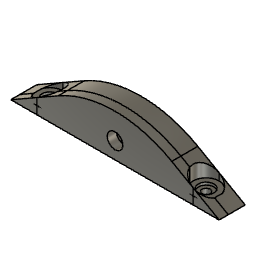
bearingholder (Autodesk Fusion 360 design; units mm, degrees)
Autodesk Fusion 360 part; units mm, degrees
form "フォーム1" [no effect]
sketch "スケッチ1" plane through (0, 0, 0) normal (0, 0, 1) x (1, 0, 0)
  line L0 (0, 0) -> (80, 0)
  line L1 (80, 0) -> (80, 5)
  line L2 (80, 5) -> (0, 5)
  line L3 (0, 5) -> (0, 0)
  circle A0 centre (10, 2.5) radius 1.5
  circle A1 centre (10, 2.5) radius 5
  circle A2 centre (10, 2.5) radius 3
  circle A3 centre (70, 2.5) radius 5
  circle A4 centre (70, 2.5) radius 3
  circle A5 centre (70, 2.5) radius 1.5
  constraint horizontal L0
  constraint vertical L1
  constraint horizontal L2
  constraint vertical L3
  constraint coincident L0.start L3.end
  constraint concentric A0 A1
  constraint concentric A1 A2
extrude "押し出し1" add sketch "スケッチ1" along normal blind 2 contours L0 L2 L3 A1 | L0 L2 A2 | L0 A2 | L0 L2 A1 A3 | L2 A2 | L0 L2 A4 | L0 A4 | L0 L1 L2 A3 | L2 A4 makes body 1 at (48.338, 2.3754, 0) makes body 2 at (78.3287, 2.6246, 2) makes body 3 at (12.9963, 2.3505, 0.6667) makes body 4 at (69.627, 5.4767, 0.6667) makes body 5 at (1.6713, 2.6246, 0)
extrude "押し出し2" add sketch "スケッチ1" along normal blind 20 contours L0 L2 A1 A2 | L0 A1 A2 | L2 A1 A2 | L0 L2 A1 A2 | L0 L2 A3 A4 | L0 A3 A4 | L2 A3 A4 | L0 L2 A3 A4 bodies 1 2 3 4 5
extrude "押し出し3" add 3 faces at (48.3427, 2.5, 2) (78.3333, 2.5, 2) (1.6713, 2.6246, 2) along direction (0, 0, 1) blind 30 on bodies 1 bodies 1
sketch "スケッチ2" plane through (0, 0, 0) normal (0, -1, 0) x (1, 0, 0)
  line L0 (14.3301, 0) -> (65.6699, 0)
  line L1 (65.6699, 0) -> (65.6699, 20)
  line L2 (65.6699, 20) -> (65.6699, 32)
  line L3 (65.6699, 32) -> (14.3301, 32)
  line L4 (14.3301, 32) -> (14.3301, 20)
  line L5 (14.3301, 20) -> (14.3301, 0)
  line L6 (0, 0) -> (35.0031, 20)
  line L7 (45, 20) -> (80, 0)
  arc A0 (45, 20) -> (35.0031, 20) centre (40.0016, 11.252) ccw
  line L8 (0, 0) -> (80.0579, 0)
  line L9 (80.0579, 0) -> (80.0579, 32)
  line L10 (80.0579, 32) -> (0, 32)
  line L11 (0, 32) -> (0, 0)
  constraint coincident L6.start L8.start
  constraint tangent L6 A0
  constraint horizontal L8
  constraint vertical L9
  constraint horizontal L10
  constraint vertical L11
extrude "押し出し4" cut sketch "スケッチ2" along normal mid plane 20 contours L4 L5 L6 L10 L11 | L1 L2 L3 L4 L5 L6 L7 A0 L10 | L1 L2 L7 L8 L9 L10 bodies 1
sketch "スケッチ3" plane through (0, 0, 0) normal (0, -1, 0) x (1, 0, 0)
  line L0 (35.0031, 20) -> (14.3301, 8.1879)
  line L1 (14.3301, 8.1879) -> (14.3301, 0)
  line L2 (14.3301, 0) -> (65.6699, 0)
  line L3 (65.6699, 0) -> (65.6699, 8.1886)
  line L4 (65.6699, 8.1886) -> (45, 20)
  arc A0 (45, 20) -> (35.0031, 20) centre (40.0016, 11.252) ccw
  line L5 (40.0016, 21.3273) -> (40.0016, 0)
  line L6 (40.0016, 0) -> (40.0016, 6.35)
  circle A1 centre (40.0016, 6.35) radius 5
  dimension "d9" = 6.35
  dimension "d10" = 10
  constraint midpoint A0 L5.start
  constraint vertical L5
  constraint perpendicular L2 L6
  constraint coincident L6.end A1.centre
  measures "d9" distance of L5.end L6.end
  measures "d10" diameter of A1
extrude "押し出し5" cut sketch "スケッチ3" against normal blind 21 contours L5 L6 A1 | L5 L6 A1 bodies 1
extrude "押し出し6" cut 3 faces at (28.2767, 0, 12.2358) (76.2201, 0, 1.08) (3.7799, 0, 1.0799) along direction (0, 1, 0) blind 1 on bodies 1 bodies 1
extrude "押し出し7" cut 3 faces at (28.2767, 5, 12.2358) (76.2201, 5, 1.08) (3.7799, 5, 1.0799) along direction (0, -1, 0) blind 1 on bodies 1 bodies 1
extrude "押し出し8" add sketch "スケッチ1" along normal blind 16 contours L0 L2 A1 A2 | L0 A1 A2 | L2 A1 A2 | L0 L2 A1 A2 bodies 1
extrude "押し出し9" add sketch "スケッチ1" along normal blind 17 contours L0 L2 A3 A4 | L0 A3 A4 | L2 A3 A4 | L0 L2 A3 A4 bodies 1
extrude "押し出し10" cut sketch "スケッチ2" along normal mid plane 28 contours L4 L5 L6 L10 L11 | L1 L2 L3 L4 L5 L6 L7 A0 L10 | L1 L2 L7 L8 L9 L10 bodies 1
extrude "押し出し11" add sketch "スケッチ1" along normal blind 15 contours L0 L2 A3 A4 | L0 A3 A4 | L2 A3 A4 | L0 L2 A3 A4 bodies 1
extrude "押し出し12" cut 1 faces at (68.0578, -1.3609, 15) along direction (0, 0, -1) blind 12 on bodies 1 bodies 1
sketch "スケッチ4" plane through (0, 0, 3) normal (0, 0, 1) x (-1, 0, 0)
  circle A0 centre (-70, -2.5) radius 3
  arc A1 (-65.2303, -4) -> (-65.2303, -1) centre (-70, -2.5) ccw
  arc A2 (-65.2303, -1) -> (-65.2303, -4) centre (-70, -2.5) ccw
  line L0 (-65.2303, -4) -> (-67.4019, -4)
  line L1 (-65.2303, -1) -> (-67.4019, -1)
  constraint coincident A1.start A2.end
  constraint coincident A0 L0.end
  constraint horizontal L0
  constraint coincident A1.end A2.start
  constraint coincident A0 L1.end
  constraint parallel L0 L1
extrude "押し出し13" add sketch "スケッチ4" along normal blind 6 contours A0 A1 L0 L1 bodies 1
extrude "押し出し14" cut sketch "スケッチ2" against normal blind 30 contours L1 L2 L3 L4 L5 L6 L7 A0 L10 | L1 L2 L7 L8 L9 L10 bodies 1
extrude "押し出し15" add sketch "スケッチ1" along normal blind 13 contours L0 L2 A1 A2 | L0 A1 A2 | L2 A1 A2 | L0 L2 A1 A2 bodies 1
extrude "押し出し16" cut 1 faces at (14.3147, 2.7484, 13) along direction (0, 0, -1) blind 10 on bodies 1 bodies 1
sketch "スケッチ5" plane through (0, 0, 3) normal (0, 0, 1) x (-1, 0, 0)
  circle A0 centre (-10, -2.5) radius 3
  arc A1 (-14.7697, -4) -> (-14.7697, -1) centre (-10, -2.5) ccw
  arc A2 (-14.7697, -1) -> (-14.7697, -4) centre (-10, -2.5) ccw
  line L0 (-14.7697, -4) -> (-12.5981, -4)
  line L1 (-14.7697, -1) -> (-12.5981, -1)
  constraint coincident A1.start A2.end
  constraint coincident A0 L0.end
  constraint horizontal L0
  constraint coincident A1.end A2.start
  constraint coincident A0 L1.end
  constraint parallel L0 L1
extrude "押し出し17" add sketch "スケッチ5" along normal blind 8 contours A0 A2 L0 L1 bodies 1
extrude "押し出し18" cut sketch "スケッチ2" against normal blind 13 contours L4 L5 L6 L10 L11 | L1 L2 L3 L4 L5 L6 L7 A0 L10 bodies 1
copy_body "ボディ -> コンポーネント1" bodies 1 removing the originals makes body 6 in component "Component'"
sketch "スケッチ6" plane through (0, 1, 0) normal (0, -1, 0) x (1, 0, 0)
  line L0 (35.0031, 20) -> (12.5981, 7.1983)
  line L1 (12.5981, 7.1983) -> (12.5981, 3)
  line L2 (12.5981, 3) -> (14.7697, 3)
  line L3 (14.7697, 3) -> (14.7697, 0)
  line L4 (14.7697, 0) -> (65.2303, 0)
  line L5 (65.2303, 0) -> (65.2303, 3)
  line L6 (65.2303, 3) -> (67.4019, 3)
  line L7 (67.4019, 3) -> (67.4019, 7.1989)
  line L8 (67.4019, 7.1989) -> (45, 20)
  arc A0 (45, 20) -> (35.0031, 20) centre (40.0016, 11.252) ccw
  circle A1 centre (40.0016, 6.35) radius 5
  line L9 (12.5981, 7.1983) -> (23.8006, 13.5991)
  line L10 (18.1993, 10.3987) -> (12.5981, 7.1983)
  line L11 (67.4019, 7.1989) -> (56.201, 13.5995)
  line L12 (61.8014, 10.3992) -> (67.4019, 7.1989)
  arc A2 (61.8014, 10.3992) -> (18.1993, 10.3987) centre (40.0008, -27.7573) ccw
  constraint coincident L0.end L1.start
  constraint midpoint L0 L9.end
  constraint midpoint L9 L10.start
  constraint coincident L7.end L8.start
  constraint midpoint L8 L11.end
  constraint midpoint L11 L12.start
  constraint tangent L10 A2
extrude "押し出し1'" cut sketch "スケッチ6" against normal blind 30 contours L0 L8 A0 L9 L11 A2 bodies 6 in component "Component'"
sketch "スケッチ7" plane through (0, 0, 0) normal (0, 0, -1) x (1, 0, 0)
  circle A0 centre (70, -2.5) radius 1.5
  line L0 (14.7697, -4) -> (65.2303, -4)
  arc A1 (65.2303, -4) -> (74.7697, -4) centre (70, -2.5) ccw
  line L1 (74.7697, -4) -> (80, -4)
  line L2 (80, -4) -> (80, -1)
  line L3 (80, -1) -> (74.7697, -1)
  arc A2 (74.7697, -1) -> (65.2303, -1) centre (70, -2.5) ccw
  line L4 (65.2303, -1) -> (14.7697, -1)
  arc A3 (14.7697, -1) -> (5.2303, -1) centre (10, -2.5) ccw
  line L5 (5.2303, -1) -> (0, -1)
  line L6 (0, -1) -> (0, -4)
  line L7 (0, -4) -> (5.2303, -4)
  arc A4 (5.2303, -4) -> (14.7697, -4) centre (10, -2.5) ccw
  circle A5 centre (10, -2.5) radius 1.5
  line L8 (10, 2.5) -> (70, 2.5)
  line L9 (70, 2.5) -> (80, 2.5)
  line L10 (80, -1) -> (80, 2.5)
  line L11 (10, 2.5) -> (0, 2.5)
  line L12 (0, 2.5) -> (0, -1)
  constraint midpoint A3 L8.start
  constraint midpoint A2 L8.end
  constraint tangent A2 L9
  constraint parallel L8 L9
  constraint coincident L2.end L3.start
  constraint perpendicular L9 L10
  constraint tangent A3 L11
  constraint perpendicular L10 L11
  constraint coincident L5.end L6.start
  constraint perpendicular L5 L12
extrude "押し出し19" add sketch "スケッチ7" against normal blind 18 separate body contours A3 L5 L11 L12 | L3 A2 L9 L10 | A2 L4 A3 L8 makes body 7
sketch "スケッチ8" plane through (0, 4, 0) normal (0, 1, 0) x (-1, 0, 0)
  arc A0 (-18.1993, 10.3987) -> (-61.8014, 10.3992) centre (-40.0008, -27.7573) ccw
  line L0 (-61.8014, 10.3992) -> (-67.4019, 7.1989)
  line L1 (-67.4019, 7.1989) -> (-67.4019, 3)
  line L2 (-67.4019, 3) -> (-65.2303, 3)
  line L3 (-65.2303, 3) -> (-65.2303, 0)
  line L4 (-65.2303, 0) -> (-14.7697, 0)
  line L5 (-14.7697, 0) -> (-14.7697, 3)
  line L6 (-14.7697, 3) -> (-12.5981, 3)
  line L7 (-12.5981, 3) -> (-12.5981, 7.1983)
  line L8 (-12.5981, 7.1983) -> (-18.1993, 10.3987)
  circle A1 centre (-40.0016, 6.35) radius 5
  line L9 (0, 0) -> (0, 18)
  line L10 (0, 18) -> (-80, 18)
  line L11 (-80, 18) -> (-80, 0)
  line L12 (-80, 0) -> (0, 0)
  line L13 (-61.8014, 10.3992) -> (-80, 0)
  line L14 (0, 0) -> (-18.1993, 10.3987)
  arc A2 (-18.1993, 10.3987) -> (-61.8014, 10.3992) centre (-40.0008, -27.7573) ccw
  constraint coincident L9.start L12.end
  constraint perpendicular L6 L9
  constraint perpendicular L7 L10
  constraint perpendicular L10 L11
  constraint perpendicular L9 L12
  constraint coincident A0.end L0.start
  constraint coincident A0.start L8.end
  constraint tangent L14 A2
extrude "押し出し20" cut sketch "スケッチ8" against normal blind 11 contours A0 L0 L8 L9 L10 L11 L13 L14 A2 bodies 7
extrude "押し出し2'" add 1 faces at (74.1667, 2.5, 3) along direction (0, 0, 1) blind 6 on bodies 6 bodies 6 in component "Component'"
sketch "スケッチ9" plane through (0, 0, 9) normal (0, 0, 1) x (-1, 0, 0)
  line L0 (-74.75, -0.9388) -> (-74.75, -4.0612)
  arc A0 (-74.75, -4.0612) -> (-65.2303, -4) centre (-70, -2.5) ccw
  line L1 (-65.2303, -4) -> (-67.4019, -4)
  arc A1 (-67.4019, -1) -> (-67.4019, -4) centre (-70, -2.5) ccw
  line L2 (-67.4019, -1) -> (-65.2303, -1)
  arc A2 (-65.2303, -1) -> (-74.75, -0.9388) centre (-70, -2.5) ccw
  circle A3 centre (-70, -2.5) radius 5
  circle A4 centre (-70, -2.5) radius 3
  dimension "d47" = 10
  dimension "d48" = 6
  constraint concentric A0 A3
  constraint concentric A0 A4
  measures "d47" diameter of A3
  measures "d48" diameter of A4
extrude "押し出し3'" cut sketch "スケッチ9" against normal blind 6 contours L0 A0 L1 A1 L2 A2 A3 A4 | L0 A3 | L1 L2 A3 A4 bodies 6 in component "Component'"
extrude "押し出し4'" add 1 faces at (5.8364, 2.4253, 3) along direction (0, 0, 1) blind 6 on bodies 6 bodies 6 in component "Component'"
sketch "スケッチ10" plane through (0, 0, 9) normal (0, 0, 1) x (-1, 0, 0)
  line L0 (-5.2505, -4.0627) -> (-5.2505, -0.9373)
  arc A0 (-5.2505, -0.9373) -> (-14.7697, -1) centre (-10, -2.5) ccw
  line L1 (-14.7697, -1) -> (-12.5981, -1)
  arc A1 (-12.5981, -4) -> (-12.5981, -1) centre (-10, -2.5) ccw
  line L2 (-12.5981, -4) -> (-14.7697, -4)
  arc A2 (-14.7697, -4) -> (-5.2505, -4.0627) centre (-10, -2.5) ccw
  circle A3 centre (-10, -2.5) radius 3
  circle A4 centre (-10, -2.5) radius 5
  dimension "d53" = 6
  dimension "d54" = 10
  constraint concentric A0 A3
  constraint concentric A3 A4
  measures "d53" diameter of A3
  measures "d54" diameter of A4
extrude "押し出し5'" cut sketch "スケッチ10" against normal blind 6 contours L0 A0 L1 A1 L2 A2 A3 A4 | L0 A4 | L1 L2 A3 A4 bodies 6 in component "Component'"
sketch "スケッチ11" plane through (0, 4, 0) normal (0, 1, 0) x (-1, 0, 0)
  line L0 (-14.7697, 0) -> (-14.7697, 3)
  line L1 (-14.7697, 3) -> (-14.7697, 8.4391)
  line L2 (-14.7697, 8.4391) -> (-18.1993, 10.3987)
  arc A0 (-18.1993, 10.3987) -> (-61.8014, 10.3992) centre (-40.0008, -27.7573) ccw
  line L3 (-61.8014, 10.3992) -> (-65.2303, 8.4398)
  line L4 (-65.2303, 8.4398) -> (-65.2303, 3)
  line L5 (-65.2303, 3) -> (-65.2303, 0)
  line L6 (-65.2303, 0) -> (-14.7697, 0)
  circle A1 centre (-40.0016, 6.35) radius 5
  circle A2 centre (-40.0016, 6.35) radius 5
  dimension "d57" = 10
  constraint concentric A1 A2
  measures "d57" diameter of A2
extrude "押し出し21" cut sketch "スケッチ11" against normal blind 10 contours A1 A2 bodies 7
sketch "スケッチ12" plane through (0, 4, 0) normal (0, 1, 0) x (-1, 0, 0)
  line L0 (-14.7697, 0) -> (-14.7697, 3)
  line L1 (-14.7697, 3) -> (-14.7697, 8.4391)
  line L2 (-14.7697, 8.4391) -> (-18.1993, 10.3987)
  arc A0 (-18.1993, 10.3987) -> (-61.8014, 10.3992) centre (-40.0008, -27.7573) ccw
  line L3 (-61.8014, 10.3992) -> (-65.2303, 8.4398)
  line L4 (-65.2303, 8.4398) -> (-65.2303, 3)
  line L5 (-65.2303, 3) -> (-65.2303, 0)
  line L6 (-65.2303, 0) -> (-14.7697, 0)
  circle A1 centre (-40.0016, 6.35) radius 5
  line L7 (-80, 0) -> (-65.2303, 8.4398)
  line L8 (-14.7697, 8.4391) -> (0, 0)
  line L9 (-80, 0) -> (0, 0)
  constraint coincident L3.end L4.start
  constraint parallel L3 L7
  constraint coincident L1.end L2.start
  constraint coincident L8.end L9.end
  constraint parallel L6 L9
extrude "押し出し6'" add sketch "スケッチ12" along normal blind 3.5 bodies 6 in component "Component'"
sketch "スケッチ13" plane through (0, 0, 3) normal (0, 0, 1) x (-1, 0, 0)
  line L0 (-74.75, -4) -> (-72.5981, -4)
  arc A0 (-67.4019, -4) -> (-72.5981, -4) centre (-70, -2.5) ccw
  line L1 (-67.4019, -4) -> (-65.2303, -4)
  arc A1 (-65.2303, -4) -> (-65.2303, -1) centre (-70, -2.5) ccw
  arc A2 (-65.2303, -1) -> (-74.75, -0.9388) centre (-70, -2.5) ccw
  line L2 (-74.75, -0.9388) -> (-74.75, -4)
  circle A3 centre (-70, -2.5) radius 5
  circle A4 centre (-70, -2.5) radius 3
  line L3 (-74.75, -4) -> (-74.7697, -4)
  dimension "d62" = 10
  dimension "d63" = 6
  constraint concentric A0 A3
  constraint concentric A3 A4
  constraint coincident L0.start L2.end
  constraint coincident A3 L3.end
  constraint perpendicular L2 L3
  measures "d62" diameter of A3
  measures "d63" diameter of A4
extrude "押し出し7'" cut sketch "スケッチ13" along normal blind 10 contours L0 A0 L1 A1 A2 L2 A3 A4 | L0 L1 A3 A4 L3 bodies 6 in component "Component'"
sketch "スケッチ14" plane through (0, 0, 2) normal (0, 0, 1) x (-1, 0, 0)
  line L0 (-72.5981, -4) -> (-70, -4)
  circle A0 centre (-70, -2.5) radius 1.5
  line L1 (-70, -4) -> (-67.4019, -4)
  arc A1 (-67.4019, -4) -> (-72.5981, -4) centre (-70, -2.5) ccw
  circle A2 centre (-70, -2.5) radius 3
  circle A3 centre (-70, -2.5) radius 1.5
  constraint concentric A0 A2
  constraint concentric A2 A3
extrude "押し出し8'" cut sketch "スケッチ14" along normal blind 6.5 bodies 6 in component "Component'"
sketch "スケッチ15" plane through (0, 0, 3) normal (0, 0, 1) x (-1, 0, 0)
  line L0 (-7.4019, -4) -> (-5.2505, -4)
  line L1 (-5.2505, -4) -> (-5.2505, -0.9373)
  arc A0 (-5.2505, -0.9373) -> (-14.7697, -1) centre (-10, -2.5) ccw
  arc A1 (-14.7697, -1) -> (-14.7697, -4) centre (-10, -2.5) ccw
  line L2 (-14.7697, -4) -> (-12.5981, -4)
  arc A2 (-7.4019, -4) -> (-12.5981, -4) centre (-10, -2.5) ccw
  circle A3 centre (-10, -2.5) radius 5
  circle A4 centre (-10, -2.5) radius 3
  line L3 (-5.2505, -4) -> (-5.2303, -4)
  constraint concentric A0 A3
  constraint concentric A3 A4
  constraint coincident L0.end L1.start
  constraint coincident A3 L3.end
  constraint perpendicular L1 L3
extrude "押し出し9'" cut sketch "スケッチ15" along normal blind 7.5 contours L0 L1 A0 A1 L2 A2 A3 A4 | L0 L2 A3 A4 L3 bodies 6 in component "Component'"
sketch "スケッチ16" plane through (0, 0, 2) normal (0, 0, 1) x (-1, 0, 0)
  line L0 (-10, -4) -> (-7.4019, -4)
  arc A0 (-7.4019, -4) -> (-12.5981, -4) centre (-10, -2.5) ccw
  line L1 (-12.5981, -4) -> (-10, -4)
  circle A1 centre (-10, -2.5) radius 1.5
  circle A2 centre (-10, -2.5) radius 3
  circle A3 centre (-10, -2.5) radius 1.5
  dimension "d70" = 6
  constraint concentric A0 A2
  constraint concentric A2 A3
  measures "d70" diameter of A2
extrude "押し出し10'" cut sketch "スケッチ16" along normal blind 5.5 bodies 6 in component "Component'"
sketch "スケッチ17" plane through (0, -2.5, 0) normal (0, -1, 0) x (1, 0, 0)
  circle A0 centre (40.0016, 6.35) radius 5
  line L0 (70, 5.7143) -> (61.8014, 10.3992)
  arc A1 (61.8014, 10.3992) -> (18.1993, 10.3987) centre (40.0008, -27.7573) ccw
  line L1 (18.1993, 10.3987) -> (10, 5.7138)
  line L2 (10, 5.7138) -> (10, 0)
  line L3 (10, 0) -> (70, 0)
  line L4 (70, 0) -> (70, 5.7143)
  circle A2 centre (40.0016, 6.35) radius 5
  circle A3 centre (40.0016, 6.35) radius 2.5
  dimension "d73" = 5
  constraint concentric A0 A2
  constraint concentric A2 A3
  measures "d73" diameter of A3
extrude "押し出し22" add sketch "スケッチ17" against normal blind 3.5 separate body contours A0 A2 makes body 8
sketch "スケッチ18" plane through (0, 7.5, 0) normal (0, 1, 0) x (-1, 0, 0)
  circle A0 centre (-40.0016, 6.35) radius 5
  line L0 (0, 0) -> (-10, 5.7138)
  line L1 (-10, 5.7138) -> (-10, 3)
  line L2 (-10, 3) -> (-10, 5.7138)
  line L3 (-10, 5.7138) -> (-18.1993, 10.3987)
  arc A1 (-18.1993, 10.3987) -> (-61.8014, 10.3992) centre (-40.0008, -27.7573) ccw
  line L4 (-61.8014, 10.3992) -> (-70, 5.7143)
  line L5 (-70, 5.7143) -> (-70, 3)
  line L6 (-70, 3) -> (-70, 5.7143)
  line L7 (-70, 5.7143) -> (-80, 0)
  line L8 (-80, 0) -> (0, 0)
  circle A2 centre (-40.0016, 6.35) radius 5
  circle A3 centre (-40.0016, 6.35) radius 3
  dimension "d76" = 10
  dimension "d77" = 6
  constraint concentric A0 A2
  constraint concentric A2 A3
  measures "d76" diameter of A2
  measures "d77" diameter of A3
extrude "押し出し23" add sketch "スケッチ18" against normal blind 3.5 separate body contours A0 A2 makes body 9
sketch "スケッチ19" plane through (0, -2.5, 0) normal (0, -1, 0) x (1, 0, 0)
  circle A0 centre (40.0016, 6.35) radius 2.5
  circle A1 centre (40.0016, 6.35) radius 5
  circle A2 centre (40.0016, 6.35) radius 3
  dimension "d80" = 6
  constraint concentric A0 A2
  measures "d80" diameter of A2
extrude "押し出し24" cut sketch "スケッチ19" against normal blind 3.5 contours A2 bodies 8
extrude "押し出し25" cut 1 faces at (44.3051, -2.5, 5.9526) along direction (0, 1, 0) blind 19 on bodies 8 bodies 8 9
sketch "スケッチ20" plane through (0, -2.5, 0) normal (0, -1, 0) x (1, 0, 0)
  circle A0 centre (40.0016, 6.35) radius 5
  line L0 (70, 5.7143) -> (61.8014, 10.3992)
  arc A1 (61.8014, 10.3992) -> (18.1993, 10.3987) centre (40.0008, -27.7573) ccw
  line L1 (18.1993, 10.3987) -> (10, 5.7138)
  line L2 (10, 5.7138) -> (10, 0)
  line L3 (10, 0) -> (70, 0)
  line L4 (70, 0) -> (70, 5.7143)
  circle A2 centre (40.0016, 6.35) radius 5.3
  dimension "d85" = 10.6
  constraint concentric A0 A2
  measures "d85" diameter of A2
extrude "押し出し26" cut sketch "スケッチ20" against normal blind 11 contours A2 bodies 7
extrude "押し出し11'" cut sketch "スケッチ20" against normal blind 11 contours A2 bodies 6 in component "Component'"
sketch "スケッチ21" plane through (0, -2.5, 0) normal (0, -1, 0) x (1, 0, 0)
  circle A0 centre (40.0016, 6.35) radius 5.3
  line L0 (70, 5.7143) -> (61.8014, 10.3992)
  arc A1 (61.8014, 10.3992) -> (18.1993, 10.3987) centre (40.0008, -27.7573) ccw
  line L1 (18.1993, 10.3987) -> (10, 5.7138)
  line L2 (10, 5.7138) -> (10, 0)
  line L3 (10, 0) -> (70, 0)
  line L4 (70, 0) -> (70, 5.7143)
  circle A2 centre (40.0016, 6.35) radius 3
  dimension "d90" = 6
  constraint concentric A0 A2
  measures "d90" diameter of A2
extrude "押し出し27" add sketch "スケッチ21" against normal blind 3.5 contours A0 bodies 8 7 9
sketch "スケッチ22" plane through (0, 7.5, 0) normal (0, 1, 0) x (-1, 0, 0)
  circle A0 centre (-40.0016, 6.35) radius 5.3
  line L0 (0, 0) -> (-10, 5.7138)
  line L1 (-10, 5.7138) -> (-10, 3)
  line L2 (-10, 3) -> (-10, 5.7138)
  line L3 (-10, 5.7138) -> (-18.1993, 10.3987)
  arc A1 (-18.1993, 10.3987) -> (-61.8014, 10.3992) centre (-40.0008, -27.7573) ccw
  line L4 (-61.8014, 10.3992) -> (-70, 5.7143)
  line L5 (-70, 5.7143) -> (-70, 3)
  line L6 (-70, 3) -> (-70, 5.7143)
  line L7 (-70, 5.7143) -> (-80, 0)
  line L8 (-80, 0) -> (0, 0)
  circle A2 centre (-40.0016, 6.35) radius 3
  dimension "d93" = 6
  constraint concentric A0 A2
  measures "d93" diameter of A2
extrude "押し出し28" add sketch "スケッチ22" against normal blind 3.5 separate body contours A0 makes body 10
component "Component'" placed x (1, 0, 0) y (0, 1, 0) z (0, 0, 1) at (0, 0, 0)
